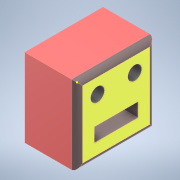
# Autodesk Inventor part: face
Saved by Autodesk Inventor 2022 (Build 260153070, 153G)
## iProperties
Created: 2021-07-03
Part Number: face
Material: PBT Plastic
Document SubType Name: Modeling
Designer: AKASH ARYAN
Density: 1.31 g/cm^3
Appearance: Smooth - White
Author: AKASH ARYAN
Autodesk Inventor part; units mm, degrees
ref_plane "YZ Plane" through (0, 0, 0) normal (1, 0, 0) x (0, 1, 0)
ref_plane "XZ Plane" through (0, 0, 0) normal (0, 1, 0) x (-1, 0, 0)
ref_plane "XY Plane" through (0, 0, 0) normal (0, 0, 1) x (1, 0, 0)
sketch "Sketch1" plane through (0, 0, 0) normal (1, 0, 0) x (0, 1, 0)
  line L0 (0, 0) -> (-114.3, 0)
  line L1 (-114.3, 0) -> (-114.3, -114.3)
  line L2 (-114.3, -114.3) -> (0, -114.3)
  line L3 (0, -114.3) -> (0, 0)
  dimension "d0" = 114.3
  dimension "d1" = 114.3
  constraints: 8 end point, 2 parallel, 1 horizontal, 1 perpendicular
  measures "d0" distance of L2.end L1.end
  measures "d1" distance of L1.end L0.end
extrude "Extrusion1" add sketch "Sketch1" along normal blind 76.2
sketch "Sketch2" plane through (76.2, 0, 0) normal (1, 0, 0) x (0, 0, -1)
  circle A0 centre (30, -30) radius 10
  circle A1 centre (84.3, -30) radius 10
  line L0 (25.4, -68.9) -> (88.9, -68.9)
  line L1 (88.9, -68.9) -> (88.9, -88.9)
  line L2 (88.9, -88.9) -> (25.4, -88.9)
  line L3 (25.4, -88.9) -> (25.4, -68.9)
  line L4 (114.3, 0) -> (0, 0) projected
  line L5 (114.3, -114.3) -> (114.3, 0) projected
  line L6 (0, 0) -> (0, -114.3) projected
  line L7 (0, -114.3) -> (114.3, -114.3) projected
  dimension "d4" = 20
  dimension "d5" = 20
  dimension "d6" = 63.5
  dimension "d7" = 20
  dimension "d8" = 30
  dimension "d9" = 30
  dimension "d10" = 30
  dimension "d11" = 30
  dimension "d12" = 25.4
  dimension "d13" = 25.4
  constraints: 8 end point, 2 centre point, 2 parallel, 1 horizontal, 1 perpendicular
  measures "d4" diameter of A0
  measures "d5" diameter of A1
  measures "d6" distance of L1.end L2.end
  measures "d7" distance of L0.end L1.end
  measures "d8" distance from line of L4 A0.centre
  measures "d9" distance from line of L4 A1.centre
  measures "d10" distance from line of L5 A1.centre
  measures "d11" distance from line of L6 A0.centre
  measures "d12" distance between parallel lines of L5 L1
  measures "d13" distance between parallel lines of L7 L2
extrude "Extrusion2" cut sketch "Sketch2" against normal through all contours A0 | A1 | L0 L1 L2 L3
sketch "Sketch3" plane through (76.2, 0, 0) normal (1, 0, 0) x (0, 0, -1)
  point P0 (0, 0)
fillet "Fillet2" radius 8 4 edges at (76.2, -57.15, 0) (76.2, 0, -57.15) (76.2, -114.3, -57.15) (76.2, -57.15, -114.3)
sketch "Sketch4" plane through (76.2, 0, 0) normal (1, 0, 0) x (0, 0, -1)
  point P0 (0, 0)
sketch "Sketch5" plane through (0, 0, 0) normal (-1, 0, 0) x (0, 0, 1)
  circle A0 centre (-57.15, -25.4) radius 2
  circle A1 centre (-57.15, -101.6) radius 2
  line L0 (-114.3, 0) -> (0, 0) projected
  line L1 (0, -114.3) -> (-114.3, -114.3) projected
  line L2 (-114.3, -114.3) -> (-114.3, 0) projected
  dimension "d18" = 4
  dimension "d19" = 4
  dimension "d20" = 25.4
  dimension "d21" = 12.7
  dimension "d22" = 57.15
  dimension "d23" = 57.15
  constraints: 2 centre point
  measures "d18" diameter of A0
  measures "d19" diameter of A1
  measures "d20" distance from line of L0 A0.centre
  measures "d21" distance from line of A1.centre L1
  measures "d22" distance from line of A0.centre L2
  measures "d23" distance from line of L2 A1.centre
extrude "Extrusion3" cut sketch "Sketch5" against normal blind 25.4
body "Solid1"
